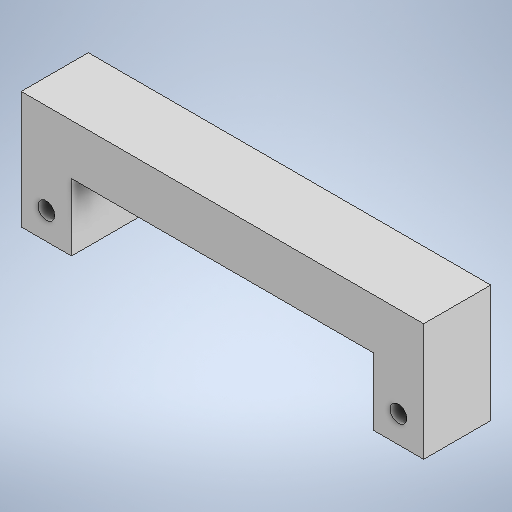
# Autodesk Inventor part: front_U_shaped_frame[1]
Saved by Autodesk Inventor 2025.2 (Build 292293000, 293)
## iProperties
Created: 2025-02-06
Part Number: front_U_shaped_frame[1]
Material: Generic
Document SubType Name: Modeling
Designer: mpava
Density: 1 g/cm^3
Appearance: Default
Author: mpava
Autodesk Inventor part; units mm, degrees
ref_plane "YZ Plane" through (0, 0, 0) normal (1, 0, 0) x (0, 1, 0)
ref_plane "XZ Plane" through (0, 0, 0) normal (0, 1, 0) x (-1, 0, 0)
ref_plane "XY Plane" through (0, 0, 0) normal (0, 0, 1) x (1, 0, 0)
sketch "Sketch1" plane through (0, 0, 0) normal (0, 0, 1) x (1, 0, 0)
  line L0 (-60, 7.5) -> (60, 7.5)
  line L1 (60, 7.5) -> (60, -7.5)
  line L2 (60, -7.5) -> (-60, -7.5)
  line L3 (-60, -7.5) -> (-60, 7.5)
  line L4 (-60, 7.5) -> (60, -7.5) construction
  line L5 (60, 7.5) -> (-60, -7.5) construction
  line L6 (-60, -7.5) -> (-45, -7.5)
  line L7 (-45, -7.5) -> (-45, -27.5)
  line L8 (-45, -27.5) -> (-60, -27.5)
  line L9 (-60, -27.5) -> (-60, -7.5)
  line L10 (60, -7.5) -> (45, -7.5)
  line L11 (45, -7.5) -> (45, -27.5)
  line L12 (45, -27.5) -> (60, -27.5)
  line L13 (60, -27.5) -> (60, -7.5)
  circle A0 centre (-52.5, -19.5) radius 2.5
  circle A1 centre (52.5, -19.5) radius 2.5
  point P0 (0, 0)
  dimension "d17" = 120
  dimension "d18" = 15
  dimension "d19" = 15
  dimension "d20" = 20
  dimension "d21" = 15
  dimension "d22" = 20
  dimension "d23" = 5
  dimension "d24" = 5
  constraints: 28 end point, 6 parallel, 3 horizontal, 3 perpendicular, 2 centre point, 2 midpoint
  measures "d17" distance of L1.end L2.end
  measures "d18" distance of L0.end L1.end
  measures "d19" distance of L7.end L8.end
  measures "d20" distance of L6.end L7.end
  measures "d21" distance of L12.end L11.end
  measures "d22" distance of L11.end L10.end
  measures "d23" diameter of A0
  measures "d24" diameter of A1
extrude "Extrusion1" add sketch "Sketch1" along normal blind 20
body "Solid1"
